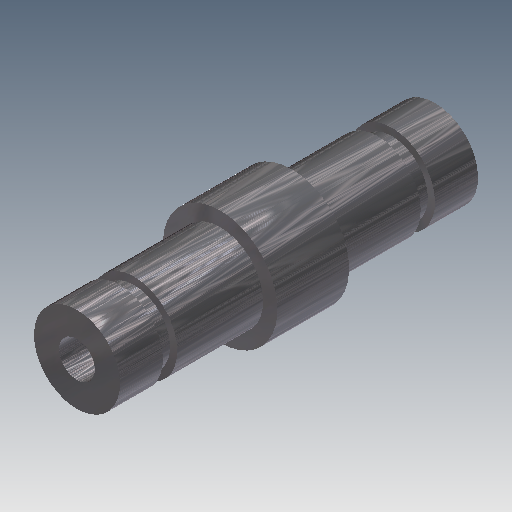
# Autodesk Inventor part: 下側ベアリング軸
Saved by Autodesk Inventor 2019.4 (Build 234330000, 330)
## iProperties
Created: 2018-08-09
Part Number: 下側ベアリング軸
Material: アルミニウム 2014-T4
Document SubType Name: Modeling
Designer: Owner
Density: 2.8 g/cm^3
Appearance: サテン
Mass: 1.89509 g
Surface Area: 8.17992 cm^2
Volume: 0.676817 cm^3
Author: Owner
Autodesk Inventor part; units mm, degrees
ref_plane "YZ Plane" through (0, 0, 0) normal (1, 0, 0) x (0, 1, 0)
ref_plane "XZ Plane" through (0, 0, 0) normal (0, 1, 0) x (-1, 0, 0)
ref_plane "XY Plane" through (0, 0, 0) normal (0, 0, 1) x (1, 0, 0)
sketch "スケッチ2" plane through (0, 0, 0) normal (1, 0, 0) x (0, 1, 0)
  line L0 (2.5, -8.5) -> (3, -8.5)
  line L1 (3, -9.5) -> (2.5, -9.5)
  line L2 (2.5, -9.5) -> (2.5, -8.5)
  line L3 (3, -9.5) -> (3, -12.5)
  line L4 (3, -12.5) -> (1.25, -12.5)
  line L5 (1.25, -12.5) -> (1.25, 0)
  line L6 (1.25, 0) -> (4, 0)
  line L7 (4, 0) -> (4, -2.5)
  line L8 (4, -2.5) -> (3, -2.5)
  line L9 (3, -2.5) -> (3, -8.5)
  line L10 (0, -15) -> (0, 2.5) projected
  point P0 (0, 0)
  dimension "d3" = 8.5
  dimension "d4" = 1
  dimension "d5" = 2.5
  dimension "d6" = 1.25
  dimension "d8" = 4
  dimension "d9" = 2.5
  dimension "d10" = 3
  dimension "d11" = 12.5
  constraints: 20 end point, 6 perpendicular, 3 point on line, 1 horizontal, 1 parallel, 1 vertical
  measures "d3" distance from line of L0 point (0, 0)
  measures "d4" distance of L0.end L1.start
  measures "d5" distance from line of point (0, 0) L2
  measures "d6" distance from line of point (0, 0) L5
  measures "d8" distance from line of point (0, 0) L7
  measures "d9" distance between parallel lines of L6 L8
  measures "d10" distance from line of point (0, 0) L9
  measures "d11" distance between parallel lines of L6 L4
revolve "回転1" add sketch "スケッチ2" angle 360 about axis through (0, 0, -10) along (0, 0, 1)
mirror "ミラー1" about plane through (0, 4, 0) normal (0, 0, 1) of "回転1"
sketch "スケッチ1" plane through (0, 0, 0) normal (0, 0, 1) x (1, 0, 0)
  circle A0 centre (0, 0) radius 4
  dimension "d0" = 8
  constraints: 1 centre point, 1 coincident
  measures "d0" diameter of A0
